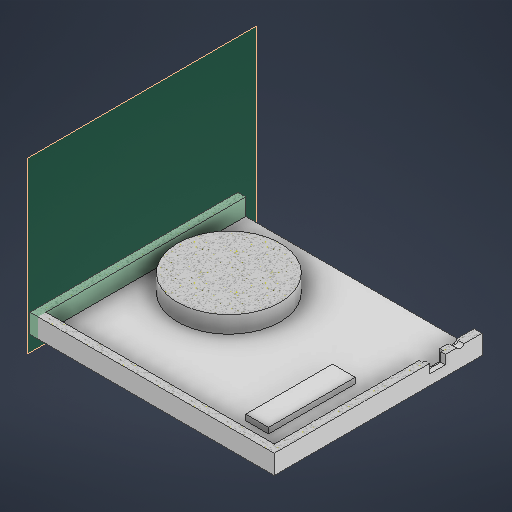
# Autodesk Inventor part: estructura_pieza1
Saved by Autodesk Inventor 2026.2 (Build 302298010, 298A)
## iProperties
Created: 2026-03-03
Part Number: estructura_pieza1
Material: Genérico
Document SubType Name: Modeling
Designer: juanm
Density: 1 g/cm^3
Appearance: Valor por defecto
Author: juanm
Autodesk Inventor part; units mm, degrees
ref_plane "YZ Plane" through (0, 0, 0) normal (1, 0, 0) x (0, 1, 0)
ref_plane "XY Plane" through (0, 0, 0) normal (0, 0, 1) x (1, 0, 0)
sketch "Boceto1" plane through (0, 0, 0) normal (1, 0, 0) x (0, 1, 0)
  line L0 (135, 82) -> (0, 82)
  line L1 (0, 82) -> (0, -100)
  line L2 (0, -100) -> (135, -100)
  line L3 (135, -100) -> (135, 82)
  line L4 (135, 82) -> (0, -100) construction
  line L5 (0, 82) -> (135, -100) construction
  point P0 (0, 0)
  point P1 (67.5, -9)
  dimension "d0" = 182
  dimension "d1" = 135
  dimension "d2" = 100
  constraints: 12 end point, 2 midpoint, 2 parallel, 1 horizontal, 1 perpendicular, 1 point on line
  measures "d0" distance of L0.end L1.end
  measures "d1" distance of L1.end L2.end
  measures "d2" distance from line of point (0, 0) L2
extrude "Extrusión1" add sketch "Boceto1" against normal blind 214
sketch "Boceto2" plane through (-214, 0, 0) normal (-1, 0, 0) x (0, 0, 1)
  line L0 (82, 135) -> (-100, 135) projected
  line L1 (-93, 2) -> (75, 2)
  line L2 (75, 2) -> (75, 135)
  line L3 (75, 135) -> (-93, 135)
  line L4 (-93, 135) -> (-93, 2)
  line L5 (-93, 2) -> (75, 135) construction
  line L6 (75, 2) -> (-93, 135) construction
  line L7 (-100, 0) -> (82, 0) projected
  line L8 (82, 0) -> (82, 135) projected
  line L9 (-100, 135) -> (-100, 0) projected
  point P0 (0, 0)
  point P1 (-9, 68.5)
  point P2 (-93, 135)
  dimension "d5" = 2
  dimension "d6" = 7
  dimension "d7" = 7
  constraints: 12 end point, 2 midpoint, 2 parallel, 1 horizontal, 1 perpendicular, 1 point on line
  measures "d5" distance between parallel lines of L7 L1
  measures "d6" distance between parallel lines of L8 L2
  measures "d7" distance between parallel lines of L9 L4
extrude "Extrusión2" cut sketch "Boceto2" against normal blind 207 contours L2 L1 L4 L0
sketch "Boceto3" plane through (0, 0, 82) normal (0, 0, 1) x (1, 0, 0)
  line L0 (-20, 0) -> (0, 0)
  line L1 (0, 0) -> (0, 10)
  line L2 (0, 10) -> (-20, 10)
  line L3 (-20, 10) -> (-20, 0)
  line L4 (-20, 0) -> (0, 10) construction
  line L5 (0, 0) -> (-20, 10) construction
  line L6 (-214, 0) -> (-194, 0)
  line L7 (-194, 0) -> (-194, 10)
  line L8 (-194, 10) -> (-214, 10)
  line L9 (-214, 10) -> (-214, 0)
  line L10 (-214, 0) -> (-194, 10) construction
  line L11 (-194, 0) -> (-214, 10) construction
  line L12 (-20, 92) -> (0, 92)
  line L13 (0, 92) -> (0, 102)
  line L14 (0, 102) -> (-20, 102)
  line L15 (-20, 102) -> (-20, 92)
  line L16 (-20, 92) -> (0, 102) construction
  line L17 (0, 92) -> (-20, 102) construction
  line L18 (-214, 0) -> (-214, 135) projected
  line L19 (0, 135) -> (0, 0) projected
  line L20 (0, 0) -> (-214, 0) projected
  line L21 (-214, 92) -> (-194, 92)
  line L22 (-194, 92) -> (-194, 102)
  line L23 (-194, 102) -> (-214, 102)
  line L24 (-214, 102) -> (-214, 92)
  line L25 (-214, 92) -> (-194, 102) construction
  line L26 (-194, 92) -> (-214, 102) construction
  line L27 (-214, 2) -> (-7, 2) projected
  point P0 (-10, 5)
  point P1 (-204, 5)
  point P2 (-10, 97)
  point P3 (-204, 97)
  point P4 (-10, 0)
  dimension "d10" = 20
  dimension "d11" = 10
  dimension "d13" = 10
  dimension "d14" = 20
  dimension "d65" = 100
  constraints: 48 end point, 9 collinear, 9 midpoint, 8 parallel, 4 horizontal, 4 perpendicular, 2 point on line
  measures "d10" distance of L6.start L6.end
  measures "d11" distance of L8.end L6.start
  measures "d13" distance of L12.end L13.end
  measures "d14" distance of L1.end L2.end
  measures "d65" distance between parallel lines of L27 L14
extrude "Extrusión3" add sketch "Boceto3" against normal blind 12 contours L3 L2 L1 L0 | L18 L23 L22 L21 | L12 L15 L14 L13 | L6 L9 L27 L7 | L27 L9 L8 L7
sketch "Sketch4" plane through (0, 0, 0) normal (1, 0, 0) x (0, 0, -1)
  line L0 (-82, 0) -> (-82, 135)
  line L1 (-100, 90) -> (-100, 60)
  line L2 (-82, 0) -> (100, 0) projected
  line L3 (-75, 60) -> (-65, 60)
  line L4 (-65, 60) -> (-65, 80)
  line L5 (-65, 80) -> (-75, 80)
  line L6 (-75, 80) -> (-75, 60)
  line L7 (-75, 60) -> (-65, 80) construction
  line L8 (-65, 60) -> (-75, 80) construction
  point P0 (0, 0)
  point P1 (-70, 70)
  point P2 (-70, 60)
  dimension "d43" = 17
  dimension "d44" = 7
  dimension "d45" = 20
  dimension "d46" = 60
  constraints: 16 end point, 3 midpoint, 2 parallel, 1 horizontal, 1 perpendicular
  measures "d43" distance between parallel lines of L0 L4
  measures "d44" distance between parallel lines of L0 L6
  measures "d45" distance from line of point (-70, 60) L5
  measures "d46" distance between parallel lines of L2 L3
extrude "Extrusion4" cut sketch "Sketch4" against normal up to next
sketch "Sketch5" plane through (-7, 0, 0) normal (-1, 0, 0) x (0, 0, 1)
  line L0 (-35, 130) -> (-25, 130)
  line L1 (-25, 130) -> (-25, 120)
  line L2 (-25, 120) -> (-35, 120)
  line L3 (-35, 120) -> (-35, 130)
  line L4 (5, 130) -> (15, 130)
  line L5 (15, 130) -> (15, 120)
  line L6 (15, 120) -> (5, 120)
  line L7 (5, 120) -> (5, 130)
  line L8 (-35, 40) -> (-25, 40)
  line L9 (-25, 40) -> (-25, 30)
  line L10 (-25, 30) -> (-35, 30)
  line L11 (-35, 30) -> (-35, 40)
  line L12 (15, 40) -> (5, 40)
  line L13 (5, 40) -> (5, 30)
  line L14 (5, 30) -> (15, 30)
  line L15 (15, 30) -> (15, 40)
  line L16 (-93, 135) -> (75, 135) projected
  line L17 (75, 135) -> (75, 102) projected
  line L18 (70, 2) -> (-93, 2) projected
  line L19 (75, 92) -> (75, 10) projected
  point P0 (0, 0)
  point P1 (-30, 130)
  point P2 (-30, 30)
  point P3 (10, 130)
  point P4 (15, 125)
  dimension "d25" = 10
  dimension "d26" = 10
  dimension "d27" = 10
  dimension "d28" = 10
  dimension "d29" = 100
  dimension "d31" = 5
  dimension "d32" = 60
  dimension "d77" = 50
  constraints: 32 end point, 8 parallel, 5 collinear, 4 horizontal, 4 midpoint, 4 perpendicular, 3 point on line
  measures "d25" distance of L1.end L2.end
  measures "d26" distance of L0.end L1.end
  measures "d27" distance of L8.end L9.end
  measures "d28" distance of L13.end L14.end
  measures "d29" distance of point (-30, 130) point (-30, 30)
  measures "d31" distance from line of L16 point (-30, 130)
  measures "d32" distance from line of L17 point (15, 125)
  measures "d77" distance between parallel lines of L5 L3
extrude "Extrusion5" add sketch "Sketch5" along normal blind 10
sketch "Sketch8" plane through (-7, 135, 75) normal (0, 0, -1) x (-1, 0, 0)
  line L0 (20, -20) -> (30, -20)
  line L1 (30, -20) -> (30, -10)
  line L2 (30, -10) -> (20, -10)
  line L3 (20, -10) -> (20, -20)
  line L4 (20, -20) -> (30, -10) construction
  line L5 (30, -20) -> (20, -10) construction
  line L6 (70, -20) -> (80, -20)
  line L7 (80, -20) -> (80, -10)
  line L8 (80, -10) -> (70, -10)
  line L9 (70, -10) -> (70, -20)
  line L10 (70, -20) -> (80, -10) construction
  line L11 (80, -20) -> (70, -10) construction
  line L12 (0, 0) -> (207, 0) projected
  line L13 (0, 0) -> (0, -33) projected
  point P0 (-7, -135)
  point P1 (25, -15)
  point P2 (75, -15)
  dimension "d47" = 10
  dimension "d48" = 10
  dimension "d49" = 10
  dimension "d50" = 10
  dimension "d51" = 50
  dimension "d52" = 10
  dimension "d53" = 20
  constraints: 24 end point, 4 midpoint, 4 parallel, 2 horizontal, 2 perpendicular, 1 point on line
  measures "d47" distance of L0.start L0.end
  measures "d48" distance of L6.start L6.end
  measures "d49" distance of L6.end L7.end
  measures "d50" distance of L2.end L0.start
  measures "d51" distance of point (75, -15) point (25, -15)
  measures "d52" distance between parallel lines of L12 L8
  measures "d53" distance between parallel lines of L13 L3
extrude "Extrusion6" add sketch "Sketch8" along normal blind 10
sketch "Sketch9" plane through (-7, 0, 0) normal (-1, 0, 0) x (0, 0, 1)
  line L0 (-68, 9) -> (-54, 9)
  line L1 (-54, 9) -> (-54, 29)
  line L2 (-54, 29) -> (-68, 29)
  line L3 (-68, 29) -> (-68, 9)
  line L4 (-68, 9) -> (-54, 29) construction
  line L5 (-54, 9) -> (-68, 29) construction
  line L6 (70, 2) -> (-93, 2) projected
  line L7 (-93, 2) -> (-93, 135) projected
  circle A0 centre (-81, 19) radius 4
  point P0 (0, 0)
  point P1 (-61, 19)
  dimension "d56" = 20
  dimension "d57" = 14
  dimension "d58" = 7
  dimension "d59" = 25
  dimension "d60" = 8
  dimension "d61" = 20
  dimension "d62" = 17
  constraints: 12 end point, 2 midpoint, 2 parallel, 1 centre point, 1 horizontal, 1 perpendicular
  measures "d56" distance of L0.end L1.end
  measures "d57" distance of L1.end L2.end
  measures "d58" distance between parallel lines of L6 L0
  measures "d59" distance between parallel lines of L7 L3
  measures "d60" diameter of A0
  measures "d61" distance of point (-61, 19) A0.centre
  measures "d62" distance from line of L6 A0.centre
extrude "Extrusion7" cut sketch "Sketch9" against normal up to next
sketch "Sketch10" plane through (-87, 115, 75) normal (-1, 0, 0) x (0, 0, 1)
  line L0 (0, 10) -> (-10, 10) projected
  arc A0 (-8, 10) -> (-2, 10) centre (-5, 8.1972) ccw
  line L1 (0, 20) -> (0, -13) projected
  point P0 (-75, -115)
  dimension "d66" = 3.5
  dimension "d67" = 2
  dimension "d68" = 2
  constraints: 2 point on circle, 2 point on line, 1 centre point
  measures "d66" radius of A0
  measures "d67" distance from line of L1 A0.end
  measures "d68" distance of L0.end A0.start
extrude "Extrusion8" cut sketch "Sketch10" against normal up to surface (60 mm away)
sketch "Sketch11" plane through (-87, 115, 75) normal (-1, 0, 0) x (0, 0, 1)
  line L0 (-10, 10) -> (-10, 0) projected
  line L1 (0, 0) -> (0, 10) projected
  arc A0 (-10, 4.322) -> (0, 4.0877) centre (-4.9301, 7.1893) ccw
  line L2 (-10, 4.322) -> (-10, 0)
  line L3 (0, 0) -> (-10, 0) projected
  line L4 (0, 0) -> (0, 4.0877)
  line L5 (-10, 4.322) -> (-10, 0)
  line L6 (0, 0) -> (0, 4.0877)
  line L7 (-10, 4.322) -> (-10, 0)
  line L8 (0, 0) -> (0, 4.0877)
  line L9 (-10, 4.322) -> (-10, 0)
  line L10 (0, 0) -> (0, 4.0877)
  point P0 (-75, -115)
  point P1 (-5, 0)
  point P2 (-5.0665, 1.3663)
  dimension "d71" = 5.8246
  dimension "d73" = 4.322
  dimension "d74" = 1.3663
  constraints: 16 end point, 5 collinear, 3 point on circle, 2 point on line, 1 centre point, 1 midpoint, 1 perpendicular
  measures "d71" radius of A0
  measures "d73" distance of L0.end L2.start
  measures "d74" vertical distance of point (-5, 0) point (-5.067, 1.366)
extrude "Extrusion9" cut sketch "Sketch11" against normal up to surface (60 mm away)
sketch "Sketch12" plane through (-214, 2, -93) normal (0, 1, 0) x (1, 0, 0)
  line L0 (162, -72) -> (182, -72)
  line L1 (182, -72) -> (182, -148)
  line L2 (182, -148) -> (162, -148)
  line L3 (162, -148) -> (162, -72)
  line L4 (162, -72) -> (182, -148) construction
  line L5 (182, -72) -> (162, -148) construction
  line L6 (207, 0) -> (207, -168) projected
  line L7 (207, -168) -> (0, -168) projected
  point P0 (214, -93)
  point P1 (172, -110)
  dimension "d78" = 76
  dimension "d79" = 20
  dimension "d80" = 25
  dimension "d81" = 20
  constraints: 12 end point, 2 midpoint, 2 parallel, 1 horizontal, 1 perpendicular
  measures "d78" distance of L2.end L0.start
  measures "d79" distance of L0.start L0.end
  measures "d80" distance between parallel lines of L6 L1
  measures "d81" distance between parallel lines of L7 L2
extrude "Extrusion10" add sketch "Sketch12" along normal blind 5
sketch "Sketch13" plane through (-214, 2, -93) normal (0, 0, 1) x (1, 0, 0)
  line L0 (214, 133) -> (0, 133) projected
  line L1 (0, 0) -> (207, 0) projected
  line L2 (0, 133) -> (207, 133)
  line L3 (207, 133) -> (207, 0)
  line L4 (207, 0) -> (0, 0)
  line L5 (0, 0) -> (0, 133)
  point P0 (214, -2)
  constraints: 8 end point, 2 parallel, 1 horizontal, 1 perpendicular
extrude "Extrusion11" cut sketch "Sketch13" against normal up to next
sketch "Sketch15" plane through (-214, 2, -100) normal (0, 1, 0) x (1, 0, 0)
  line L0 (20, -175) -> (0, -175) projected
  line L1 (0, 0) -> (0, -182) projected
  line L2 (7, -175) -> (0, -175)
  line L3 (0, -175) -> (0, 0)
  line L4 (0, 0) -> (7, 0)
  line L5 (7, 0) -> (7, -175)
  point P0 (214, -100)
  dimension "d90" = 7
  constraints: 8 end point, 2 parallel, 1 horizontal, 1 perpendicular, 1 point on line
  measures "d90" distance between parallel lines of L1 L5
extrude "Extrusion13" add sketch "Sketch15" along normal up to surface (133 mm away)
sketch "Sketch16" plane through (-194, 2, 75) normal (0, 1, 0) x (1, 0, 0)
  circle A0 centre (37.2, 110) radius 44.9
  line L0 (-13, 175) -> (-13, 0) projected
  line L1 (-13, 175) -> (187, 175) projected
  point P0 (194, 75)
  dimension "d93" = 89.8
  dimension "d94" = 50.2
  dimension "d95" = 65
  constraints: 1 centre point
  measures "d93" diameter of A0
  measures "d94" distance from line of L0 A0.centre
  measures "d95" distance from line of L1 A0.centre
extrude "Extrusion14" add sketch "Sketch16" along normal blind 15
sketch "Sketch17" plane through (-7, 0, 0) normal (-1, 0, 0) x (0, 0, 1)
  line L0 (-70, 31) -> (-52, 31)
  line L1 (-52, 31) -> (-52, 7)
  line L2 (-52, 7) -> (-70, 7)
  line L3 (-70, 7) -> (-70, 31)
  line L4 (-68, 29) -> (-54, 29) projected
  line L5 (-54, 29) -> (-54, 9) projected
  line L6 (-54, 9) -> (-68, 9) projected
  line L7 (-68, 9) -> (-68, 29) projected
  point P0 (0, 0)
  dimension "d98" = 2
  dimension "d99" = 2
  dimension "d100" = 2
  dimension "d101" = 2
  constraints: 8 end point, 2 parallel, 1 horizontal, 1 perpendicular
  measures "d98" distance between parallel lines of L0 L4
  measures "d99" distance between parallel lines of L1 L5
  measures "d100" distance between parallel lines of L6 L2
  measures "d101" distance between parallel lines of L7 L3
extrude "Extrusion15" cut sketch "Sketch17" against normal blind 3 contours L0 L1 L2 L3 | L4 L5 L6 L7
sketch "Sketch18" plane through (-7, 0, 0) normal (-1, 0, 0) x (0, 0, 1)
  circle A0 centre (-70, 57) radius 2.95
  line L0 (70, 2) -> (-100, 2) projected
  line L1 (-100, 2) -> (-100, 135) projected
  point P0 (0, 0)
  dimension "d104" = 5.9
  dimension "d105" = 55
  dimension "d106" = 30
  constraints: 1 centre point
  measures "d104" diameter of A0
  measures "d105" distance from line of L0 A0.centre
  measures "d106" distance from line of L1 A0.centre
extrude "Extrusion16" cut sketch "Sketch18" against normal up to surface (7 mm away)
sketch "Sketch19" plane through (-7, 0, 0) normal (-1, 0, 0) x (0, 0, 1)
  line L0 (-80, 59) -> (-75, 59)
  line L1 (-75, 59) -> (-75, 64)
  line L2 (-75, 64) -> (-80, 64)
  line L3 (-80, 64) -> (-80, 59)
  line L4 (-65, 59) -> (-60, 59)
  line L5 (-60, 59) -> (-60, 64)
  line L6 (-60, 64) -> (-65, 64)
  line L7 (-65, 64) -> (-65, 59)
  circle A0 centre (-70, 57) radius 2.95 projected
  point P0 (0, 0)
  dimension "d109" = 5
  dimension "d110" = 5
  dimension "d111" = 5
  dimension "d112" = 5
  dimension "d113" = 20
  dimension "d114" = 5
  dimension "d115" = 2
  constraints: 16 end point, 4 parallel, 2 horizontal, 2 perpendicular, 1 collinear
  measures "d109" distance of L0.end L1.end
  measures "d110" distance of L6.end L4.start
  measures "d111" distance of L5.end L6.end
  measures "d112" distance of L0.start L0.end
  measures "d113" distance between parallel lines of L5 L3
  measures "d114" distance from line of L7 A0.centre
  measures "d115" distance from line of A0.centre L0
extrude "Extrusion17" add sketch "Sketch19" along normal blind 3 contours L3 L2 L1 L0 | L7 L6 L5 L4
sketch "Sketch20" plane through (-7, 0, 0) normal (-1, 0, 0) x (0, 0, 1)
  circle A0 centre (-81, 19) radius 5
  circle A1 centre (-81, 19) radius 4 projected
  point P0 (0, 0)
  dimension "d118" = 1
  constraints: 1 centre point, 1 concentric
  measures "d118" radial gap between concentric circles of A0 A1
extrude "Extrusion18" cut sketch "Sketch20" against normal blind 2 contours A0 | A1
ref_plane "Work Plane1" through (-207, 135, 31.25) normal (-1, 0, 0) x (0, 0, 1)
split_face "Split1"
